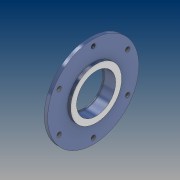
# Autodesk Inventor part: elasmaROyleman
Saved by Autodesk Inventor 2021 (Build 250183000, 183)
## iProperties
Created: 2021-01-08
Part Number: elasmaROyleman
Material: Generic
Document SubType Name: Sheet Metal
Designer: Διογενης Τσιχλακης
Density: 1 g/cm^3
Sheet Metal Rule: Default_mm
Appearance: Default
Author: Διογενης Τσιχλακης
Autodesk Inventor part; units mm, degrees
ref_plane "YZ Plane" through (0, 0, 0) normal (1, 0, 0) x (0, 1, 0)
ref_plane "XZ Plane" through (0, 0, 0) normal (0, 1, 0) x (-1, 0, 0)
sketch "Sketch1" plane through (0, 0, 0) normal (1, 0, 0) x (0, 1, 0)
  circle A0 centre (0, 0) radius 268
  circle A1 centre (0, 0) radius 203.25
  circle A2 centre (0, 0) radius 232.5
  circle A3 centre (232.5, 0) radius 12.5
  circle A4 centre (116.25, 201.3509) radius 12.5
  circle A5 centre (-116.25, 201.3509) radius 12.5
  circle A6 centre (-232.5, 0) radius 12.5
  circle A7 centre (-116.25, -201.3509) radius 12.5
  circle A8 centre (116.25, -201.3509) radius 12.5
  dimension "d2" = 465
  dimension "d0" = 536
  dimension "d1" = 406.5
  dimension "d3" = 25
  dimension "d101" = 360
  constraints: 8 centre point, 3 coincident, 1 horizontal alignment, 15 other
  measures "d0" diameter of A0
  measures "d1" diameter of A1
  measures "d3" diameter of A3
extrude "Extrusion1" add sketch "Sketch1" along normal blind 20 contours A0 | A3 A2 A8 A7 A6 A5 A4
sketch "Sketch2" plane through (0, 0, 0) normal (1, 0, 0) x (0, 1, 0)
  circle A0 centre (0, 0) radius 115
  circle A1 centre (0, 0) radius 150
  dimension "d10" = 230
  dimension "d11" = 300
  constraints: 2 centre point, 2 coincident
  measures "d10" diameter of A0
  measures "d11" diameter of A1
extrude "Extrusion2" add sketch "Sketch2" against normal mid plane 70
ref_plane "Work Plane1" through (-10, 0, 0) normal (-1, 0, 0) x (0, 0, 1)
sketch "Sketch3" plane through (-10, 0, 0) normal (-1, 0, 0) x (0, 0, 1)
  circle A0 centre (0, 0) radius 203.25
  circle A1 centre (0, 0) radius 150
  dimension "d15" = 406.5
  dimension "d16" = 300
  constraints: 2 centre point, 2 coincident
  measures "d15" diameter of A0
  measures "d16" diameter of A1
extrude "Extrusion3" add sketch "Sketch3" against normal blind 30
sketch "Sketch4" plane through (-35, 0, 0) normal (-1, 0, 0) x (0, 0, 1)
  circle A0 centre (0, 0) radius 113.4667
  circle A1 centre (0, 0) radius 111
  circle A2 centre (0, 0) radius 115
  dimension "d43" = 222
  dimension "d44" = 230
  constraints: 3 centre point, 3 coincident
  measures "d43" diameter of A1
  measures "d44" diameter of A2
extrude "Extrusion4" add sketch "Sketch4" against normal blind 6 contours A0 | A2
sketch "Sketch6" plane through (35, 0, 0) normal (1, 0, 0) x (0, 0, -1)
  circle A0 centre (0, 0) radius 150
  circle A1 centre (0, 0) radius 115
  dimension "d61" = 300
  constraints: 2 centre point
  measures "d61" diameter of A0
extrude "Extrusion6" add sketch "Sketch6" along normal blind 2.07
thread "Thread20" size "M25x2" class "6H" standard "ANSI Metric M Profile" full length
sketch "Sketch9" plane through (-10, 0, 0) normal (-1, 0, 0) x (0, 0, 1)
  circle A0 centre (0, 0) radius 203.25
  circle A1 centre (0, 0) radius 150
  constraints: 2 centre point, 2 coincident
extrude "Extrusion8" cut sketch "Sketch9" against normal up to surface (10 mm away)
thread "Thread30" size "M25x2" class "6H" standard "ANSI Metric M Profile" full length
thread "Thread31" size "M25x2" class "6H" standard "ANSI Metric M Profile" full length
thread "Thread32" size "M25x2" class "6H" standard "ANSI Metric M Profile" full length
thread "Thread33" size "M25x2" class "6H" standard "ANSI Metric M Profile" full length
thread "Thread34" size "M25x2" class "6H" standard "ANSI Metric M Profile" full length
equation "\"BendRadius\" = Thickness"
equation "\"BendReliefWidth\" = Thickness"
equation "\"BendReliefDepth\" = 0.5 * Thickness"
equation "\"CornerReliefSize\" = 4 * Thickness"
equation "\"MinimumRemnant\" = 2 * Thickness"
equation "\"TransitionRadius\" = BendRadius"
equation "\"JacobiRadiusSize\" = BendRadius"
equation "\"GapSize\" = Thickness"
equation "\"Thickness\" = 0.5"
body "Solid1"
